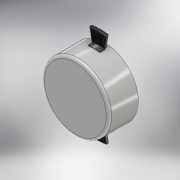
# Autodesk Inventor part: Pot
Saved by Autodesk Inventor 2020 (Build 240168000, 168)
## iProperties
Created: 2018-04-19
Part Number: Pot
Material: Generic
Document SubType Name: Modeling
Designer: PC  USER
Density: 1 g/cm^3
Appearance: Default
Author: PC  USER
Autodesk Inventor part; units mm, degrees
ref_plane "YZ Plane" through (0, 0, 0) normal (1, 0, 0) x (0, 1, 0)
ref_plane "XZ Plane" through (0, 0, 0) normal (0, 1, 0) x (-1, 0, 0)
sketch "Sketch1" plane through (0, 0, 0) normal (1, 0, 0) x (0, 1, 0)
  line L0 (0, 0) -> (87, 0)
  line L1 (87, 0) -> (87, -100)
  line L2 (87, -100) -> (0, -100)
  line L3 (0, -100) -> (0, 0)
  dimension "d0" = 100
  dimension "d1" = 87
  constraints: 8 end point, 2 parallel, 1 horizontal, 1 perpendicular
  measures "d0" distance of L0.end L1.end
  measures "d1" distance of L1.end L2.end
revolve "Revolution1" add sketch "Sketch1" angle 360 about axis through (0, 0, 0) along (0, 1, 0)
shell "Shell1" thickness 1 removed faces 1 at (-29.3636, 87, -20.1966)
sketch "Sketch2" plane through (0, 0, 0) normal (1, 0, 0) x (0, 1, 0)
  line L0 (0, 100) -> (0, -100) projected
  line L1 (87, 100) -> (87, -100) projected
  line L2 (71.5, -100) -> (55.5, -100)
  line L3 (55.5, -100) -> (55.5, -102)
  line L4 (55.5, -102) -> (71.5, -102)
  line L5 (71.5, -102) -> (71.5, -100)
  line L6 (71.5, -100) -> (69.5, -100)
  line L7 (69.5, -100) -> (69.5, -104)
  line L8 (69.5, -104) -> (71.5, -104)
  line L9 (71.5, -104) -> (71.5, -100)
  line L10 (76, -104) -> (65, -104)
  line L11 (65, -104) -> (65, -142)
  line L12 (65, -142) -> (76, -142)
  line L13 (76, -142) -> (76, -104)
  line L14 (87, -100) -> (0, -100) projected
  line L15 (-17.4, 0) -> (104.4, 0) projected
  point P0 (0, 0)
  point P1 (70.5, -104)
  point P2 (70.5, -104)
  dimension "d3" = 16
  dimension "d4" = 2
  dimension "d5" = 2
  dimension "d6" = 4
  dimension "d7" = 11
  dimension "d8" = 38
  dimension "d10" = 100
  dimension "d11" = 42
  dimension "d12" = 65
  constraints: 24 end point, 6 parallel, 3 horizontal, 3 perpendicular, 2 coincident, 2 midpoint
  measures "d3" distance of L3.end L4.end
  measures "d4" distance of L2.end L3.end
  measures "d5" distance of L8.end L7.end
  measures "d6" distance of L7.end L6.end
  measures "d7" distance of L11.end L12.end
  measures "d8" distance of L12.end L10.start
  measures "d10" distance from line of point (0, 0) L2
  measures "d11" distance between parallel lines of L12 L14
  measures "d12" distance between parallel lines of L0 L11
revolve "Revolution2" add sketch "Sketch2" angle 20.175 mid plane about axis through (0, -10, 0) along (0, 1, 0) contours L2 L7 L4 L3 | L2 L5 L4 L7 | L4 L9 L8 L7 | L8 L10 L13 L12 L11
ref_plane "Work Plane1" through (0, 0, -103) normal (0, 0, 1) x (1, 0, 0)
sketch "Sketch3" plane through (0, 0, -103) normal (0, 0, 1) x (1, 0, 0)
  line L0 (17.8655, 69.5) -> (-17.8655, 69.5) projected
  line L1 (17.8655, 55.5) -> (17.8655, 69.5) projected
  line L2 (17.8655, 55.5) -> (-17.8655, 55.5) projected
  line L3 (-17.8655, 69.5) -> (-17.8655, 55.5) projected
  line L4 (24.8716, 65) -> (-24.8716, 65) projected
  circle A0 centre (10.5, 60.5) radius 3
  circle A1 centre (-10.5, 60.5) radius 3
  line L5 (0, 104.4) -> (0, -17.4) projected
  point P0 (0, 0)
  dimension "d15" = 6
  dimension "d16" = 6
  dimension "d17" = 10.5
  dimension "d18" = 10.5
  dimension "d19" = 4.5
  dimension "d20" = 4.5
  constraints: 2 centre point
  measures "d15" diameter of A0
  measures "d16" diameter of A1
  measures "d17" distance from line of L5 A1.centre
  measures "d18" distance from line of L5 A0.centre
  measures "d19" distance from line of L4 A1.centre
  measures "d20" distance from line of L4 A0.centre
extrude "Extrusion1" add sketch "Sketch3" along normal blind 4.15 contours A0 | A1
mirror "Mirror1" about plane through (0, 0, 0) normal (0, 0, 1) of "Extrusion1", "Revolution2"
fillet "Fillet1" radius 1.8 4 edges at (7.5, 60.5, 103) (-13.5, 60.5, -103) (7.5, 60.5, -103) (-13.5, 60.5, 103)
fillet "Fillet1" radius 3.4 16 edges at (-21.5437, 76, -121.0986) (21.5437, 76, -121.0986) (-21.5437, 65, -121.0986) (21.5437, 65, -121.0986) (0, 76, -142) (0, 65, -142) (0, 76, 142) (0, 65, 142) (-21.5437, 76, 121.0986) (21.5437, 76, 121.0986) (21.5437, 65, 121.0986) (-21.5437, 65, 121.0986) (0, 76, 104) (0, 65, 104) (0, 76, -104) (0, 65, -104)
fillet "Fillet2" radius 8 2 edges at (0, 1, 99) (0, 0, 100)
ref_plane "Work Plane2" through (0, 70.5, 0) normal (0, 1, 0) x (1, 0, 0)
ref_plane "Work Plane3" through (0, 0, 130) normal (0, 0, 1) x (1, 0, 0)
ref_plane "Work Plane4" through (0, 0, -130) normal (0, 0, 1) x (1, 0, 0)
body "Solid1"
